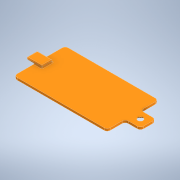
# Autodesk Inventor part: BatteryPlate
Saved by Autodesk Inventor 2021 (Build 250183000, 183)
## iProperties
Created: 2021-05-13
Part Number: BatteryPlate
Material: Generic
Document SubType Name: Modeling
Designer: ermoz
Density: 1 g/cm^3
Appearance: Default
Author: ermoz
Autodesk Inventor part; units mm, degrees
ref_plane "YZ Plane" through (0, 0, 0) normal (1, 0, 0) x (0, 1, 0)
ref_plane "XZ Plane" through (0, 0, 0) normal (0, 1, 0) x (-1, 0, 0)
ref_plane "XY Plane" through (0, 0, 0) normal (0, 0, 1) x (1, 0, 0)
sketch "Sketch1" plane through (0, 0, 0) normal (0, 1, 0) x (-1, 0, 0)
  line L0 (-30.5, -16.75) -> (30.5, -16.75)
  line L1 (30.5, -16.75) -> (30.5, 16.75)
  line L2 (30.5, 16.75) -> (-30.5, 16.75)
  line L3 (-30.5, 16.75) -> (-30.5, -16.75)
  line L4 (-30.5, -16.75) -> (30.5, 16.75) construction
  line L5 (30.5, -16.75) -> (-30.5, 16.75) construction
  point P0 (0, 0)
  dimension "d0" = 33.5
  dimension "d1" = 61
  constraints: 12 end point, 2 midpoint, 2 parallel, 1 horizontal, 1 perpendicular
  measures "d0" distance of L0.end L1.end
  measures "d1" distance of L1.end L2.end
extrude "Extrusion1" add sketch "Sketch1" along normal blind 1.5
fillet "Fillet1" radius 2 4 edges at (30.5, 0.75, 16.75) (30.5, 0.75, -16.75) (-30.5, 0.75, -16.75) (-30.5, 0.75, 16.75)
sketch "Sketch4" plane through (0, 1.5, 0) normal (0, 1, 0) x (1, 0, 0)
  line L0 (-25.5, 3.5) -> (-35.5, 3.5)
  line L1 (-35.5, 3.5) -> (-35.5, -3.5)
  line L2 (-35.5, -3.5) -> (-25.5, -3.5)
  line L3 (-25.5, -3.5) -> (-25.5, 3.5)
  line L4 (-25.5, 3.5) -> (-35.5, -3.5) construction
  line L5 (-35.5, 3.5) -> (-25.5, -3.5) construction
  line L6 (-30.5, 14.75) -> (-30.5, -14.75) projected
  point P0 (0, 0)
  point P1 (-30.5, 0)
  point P2 (-30.5, 0)
  dimension "d31" = 7
  dimension "d32" = 5
  dimension "d33" = 5
  constraints: 12 end point, 3 midpoint, 2 parallel, 1 horizontal, 1 horizontal alignment, 1 perpendicular
  measures "d31" distance of L0.end L1.end
  measures "d32" distance between parallel lines of L6 L1
  measures "d33" distance between parallel lines of L6 L3
extrude "Extrusion5" add sketch "Sketch4" along normal blind 1.5
fillet "Fillet5" radius 0.5 14 edges at (-28, 1.5, -3.5) (-25.5, 2.25, -3.5) (-25.5, 1.5, 0) (-25.5, 3, 0) (-30.5, 3, -3.5) (-33, 1.5, -3.5) (-35.5, 2.25, -3.5) (-35.5, 3, 0) (-35.5, 1.5, 0) (-35.5, 2.25, 3.5) (-33, 1.5, 3.5) (-30.5, 3, 3.5) (-28, 1.5, 3.5) (-25.5, 2.25, 3.5)
sketch "Sketch5" plane through (0, 0, 0) normal (0, -1, 0) x (1, 0, 0)
  line L0 (40.5, -5) -> (30.5, -5)
  line L1 (30.5, -5) -> (30.5, 5)
  line L2 (30.5, 5) -> (40.5, 5)
  line L3 (40.5, 5) -> (40.5, -5)
  line L4 (40.5, -5) -> (30.5, 5) construction
  line L5 (30.5, -5) -> (40.5, 5) construction
  line L6 (30.5, 14.75) -> (30.5, -14.75) projected
  point P0 (0, 0)
  point P1 (35.5, 0)
  point P2 (35.5, 0)
  dimension "d37" = 10
  dimension "d38" = 10
  constraints: 12 end point, 3 midpoint, 2 parallel, 1 collinear, 1 horizontal, 1 horizontal alignment, 1 perpendicular
  measures "d37" distance of L2.end L0.start
  measures "d38" distance of L0.start L0.end
extrude "Extrusion6" add sketch "Sketch5" against normal up to surface (1.5 mm away)
sketch "Sketch6" plane through (0, 0, 0) normal (0, -1, 0) x (1, 0, 0)
  circle A0 centre (35.5, 0) radius 1.75
  line L0 (30.5, 14.75) -> (30.5, 5) projected
  point P0 (0, 0)
  dimension "d41" = 3.5
  dimension "d42" = 5
  constraints: 1 centre point
  measures "d41" diameter of A0
  measures "d42" distance from line of L0 A0.centre
extrude "Extrusion7" cut sketch "Sketch6" against normal up to surface (1.5 mm away)
fillet "Fillet6" radius 2 4 edges at (30.5, 0.75, 5) (40.5, 0.75, 5) (40.5, 0.75, -5) (30.5, 0.75, -5)
chamfer "Chamfer1" distance 1.5 angle 45 1 edges at (33.75, 0, 0)
body "Solid1"
